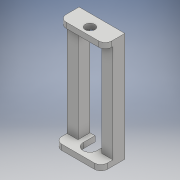
# Autodesk Inventor part: cage2table-mount-M4(top)-M6(bottom)
Saved by Autodesk Inventor 2017 (Build 210142000, 142)
## iProperties
Created: 2022-05-03
Part Number: cage2table-mount-M4(top)-M6(bottom)
Material: Generic
Document SubType Name: Modeling
Designer: Nikita
Density: 1 g/cm^3
Appearance: Default
Author: Nikita
Autodesk Inventor part; units mm, degrees
ref_plane "YZ Plane" through (0, 0, 0) normal (1, 0, 0) x (0, 1, 0)
ref_plane "XZ Plane" through (0, 0, 0) normal (0, 1, 0) x (-1, 0, 0)
ref_plane "XY Plane" through (0, 0, 0) normal (0, 0, 1) x (1, 0, 0)
sketch "Sketch1" plane through (0, 0, 0) normal (0, 0, 1) x (1, 0, 0)
  arc A0 (-3.2, 0) -> (3.2, 0) centre (0, 0) ccw
  arc A1 (-5.5, 0) -> (5.5, 0) centre (0, 0) ccw
  line L0 (-3.2, 0) -> (-5.5, 0)
  line L1 (-5.5, 0) -> (-5.5, 5.5)
  line L2 (-5.5, 5.5) -> (-3.2, 5.5)
  line L3 (-3.2, 5.5) -> (-3.2, 0)
  line L4 (3.2, 0) -> (5.5, 0)
  line L5 (5.5, 0) -> (5.5, 5.5)
  line L6 (5.5, 5.5) -> (3.2, 5.5)
  line L7 (3.2, 5.5) -> (3.2, 0)
  line L8 (-5.5, 0) -> (-5.5, 5.5)
  line L9 (-5.5, 5.5) -> (-10.5, 5.5)
  line L10 (-10.5, 5.5) -> (-10.5, 0)
  line L11 (-10.5, 0) -> (-5.5, 0)
  line L12 (5.5, 0) -> (5.5, 5.5)
  line L13 (5.5, 5.5) -> (10.5, 5.5)
  line L14 (10.5, 5.5) -> (10.5, 0)
  line L15 (10.5, 0) -> (5.5, 0)
  line L16 (10.5, 0) -> (10.5, -5.5)
  line L17 (10.5, -5.5) -> (-10.5, -5.5)
  line L18 (-10.5, -5.5) -> (-10.5, 0)
  dimension "d0" = 6.4
  dimension "d1" = 11
  dimension "d2" = 5
  dimension "d3" = 5
  constraints: 38 end point, 10 equal length, 6 perpendicular, 4 point on circle, 2 centre point, 2 coincident, 2 point on line, 2 tangent, 1 horizontal, 1 vertical
  measures "d0" diameter of A0
  measures "d1" diameter of A1
  measures "d2" distance of L9.end L1.end
  measures "d3" distance of L5.end L13.end
extrude "Extr-legs" add sketch "Sketch1" along normal blind 45 contours L11 L10 L9 L1 | L5 L13 L14 L15
extrude "Extr-base" add sketch "Sketch1" against normal blind 2.5 contours A0 L4 A1 L0 | L0 L1 L2 L3 | L7 L6 L5 L4 | L11 L10 L9 L1 | L5 L13 L14 L15
sketch "Sketch2" plane through (0, 0, 45) normal (0, 0, 1) x (1, 0, 0)
  circle A0 centre (0, 0) radius 2.2
  circle A1 centre (0, 0) radius 3.5
  line L0 (5.5, 0) -> (10.5, 0) projected
  line L1 (-10.5, 0) -> (-5.5, 0) projected
  line L2 (-10.5, 0) -> (-10.5, 5.5)
  line L3 (-10.5, 5.5) -> (10.5, 5.5)
  line L4 (10.5, 5.5) -> (10.5, 0)
  line L5 (10.5, 0) -> (2.2, 0)
  line L6 (-2.2, 0) -> (-10.5, 0)
  line L7 (-10.5, 0) -> (-10.5, -3.5)
  line L8 (-10.5, -3.5) -> (10.5, -3.5)
  line L9 (10.5, -3.5) -> (10.5, 0)
  dimension "d8" = 4.4
  dimension "d9" = 7
  constraints: 16 end point, 4 perpendicular, 3 parallel, 2 centre point, 2 coincident, 2 horizontal, 2 point on circle, 1 vertical
  measures "d8" diameter of A0
  measures "d9" diameter of A1
extrude "Extr-top" add sketch "Sketch2" along normal blind 2.5 contours L5 A1 L6 A0 | A0 L6 A1 L5 | L5 L0 L9 L8 A1 | A1 L6 L1 L2 L3 L4 L0 L5 | A1 L8 L7 L1 L6
extrude "Extrusion4" add sketch "Sketch1" against normal up to surface (2.5 mm away) contours A1 L17 L18 L11 | L15 L16 L17 A1
fillet "Fillet1" radius 3 4 edges at (10.5, -3.5, 46.25) (10.5, -5.5, -1.25) (-10.5, -3.5, 46.25) (-10.5, -5.5, -1.25)
body "Solid1"
